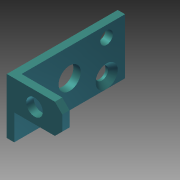
# Autodesk Inventor part: 13_0204_051
Saved by Autodesk Inventor 2012 SP1 (Build 160190100, 190)
## iProperties
Created: 2013-04-11
Part Number: 13_0204_051
Material: Default
Document SubType Name: Modeling
Designer: vogel
Density: 1 g/cm^3
Author: vogel
Autodesk Inventor part; units mm, degrees
ref_plane "YZ Plane" through (0, 0, 0) normal (1, 0, 0) x (0, 1, 0)
ref_plane "XZ Plane" through (0, 0, 0) normal (0, 1, 0) x (-1, 0, 0)
ref_plane "XY Plane" through (0, 0, 0) normal (0, 0, 1) x (1, 0, 0)
sketch "Skizze1" plane through (0, 0, 0) normal (0, 0, 1) x (1, 0, 0)
  line L0 (0, 0) -> (1.7032, 0)
  line L1 (2, 2) -> (2, 30)
  line L2 (2, 30) -> (0, 30)
  line L3 (0, 30) -> (0, 0)
  line L4 (0, 0) -> (15, 0)
  line L5 (15, 0) -> (15, 2)
  line L6 (15, 2) -> (2, 2)
  line L7 (0, 2.129) -> (0, 0)
  dimension "d0" = 30
  dimension "d1" = 15
  dimension "d2" = 2
  constraints: 16 end point, 4 parallel, 3 perpendicular, 2 horizontal
  measures "d0" distance of L2.end L0.start
  measures "d1" distance of L0.start L4.end
  measures "d2" distance of L4.end L5.end
extrude "Extrusion1" add sketch "Skizze1" along normal blind 15
sketch "Skizze2" plane through (0, 0, 0) normal (-1, 0, 0) x (0, 0, 1)
  line L0 (0, 30) -> (15, 30) projected
  line L1 (0, 0) -> (0, 30) projected
  line L2 (0, 0) -> (15, 0) projected
  line L3 (0, -6) -> (0, 36) projected
  line L4 (-3, 0) -> (18, 0) projected
  line L5 (7.5, 30) -> (7.5, 0)
  point P0 (7.5, 15)
  dimension "d5" = 30
  dimension "d6" = 7.5
  dimension "d7" = 15
  constraints: 3 midpoint, 2 end point, 1 perpendicular
  measures "d5" distance of L5.start L5.end
  measures "d6" distance between parallel lines of L5 L1
  measures "d7" distance from line of L2 point (7.5, 15)
hole "Bohrung1" at (0, 15, 7.5) direction (1, 0, 0) diameter 6 end through all
sketch "Skizze3" plane through (2, 2, 0) normal (0, 1, 0) x (1, 0, 0)
  line L0 (0, -15) -> (13, -15) projected
  line L1 (0, 0) -> (0, -15) projected
  line L2 (13, 0) -> (0, 0)
  line L3 (0, 0) -> (0, -7)
  line L4 (0, -7) -> (13, -7)
  line L5 (13, -7) -> (13, 0)
  point P0 (-2, 0)
  dimension "d15" = 8
  constraints: 8 end point, 2 parallel, 1 horizontal, 1 perpendicular, 1 point on line
  measures "d15" distance between parallel lines of L4 L0
extrude "Extrusion2" cut sketch "Skizze3" against normal through all
sketch "Skizze4" plane through (2, 0, 0) normal (1, 0, 0) x (0, 0, -1)
  line L0 (-15, 30) -> (-15, 2) projected
  line L1 (0, 30) -> (0, 0) projected
  line L2 (0, 30) -> (-15, 30) projected
  line L3 (-15, 27.5) -> (0, 27.5)
  line L4 (-15, 22) -> (0, 22)
  point P0 (-11, 25)
  point P1 (-4, 25)
  dimension "d18" = 2.5
  dimension "d19" = 8
  dimension "d20" = 5
  dimension "d21" = 5
  dimension "d22" = 4
  dimension "d23" = 4
  constraints: 4 end point, 4 point on line, 2 perpendicular
  measures "d18" distance between parallel lines of L2 L3
  measures "d19" distance between parallel lines of L2 L4
  measures "d20" distance from line of L2 point (-11, 25)
  measures "d21" distance from line of point (-4, 25) L2
  measures "d22" distance from line of point (-4, 25) L1
  measures "d23" distance from line of L0 point (-11, 25)
hole "Bohrung2" at (2, 25, 11) at (2, 25, 4) direction (-1, 0, 0) diameter 3.4 end through all
sketch "Skizze5" plane through (2, 2, 15) normal (0, 1, 0) x (1, 0, 0)
  line L0 (13, 8) -> (0, 8) projected
  line L1 (13, 8) -> (13, 0) projected
  point P0 (-2, 15)
  point P1 (5.5, 4)
  dimension "d31" = 7.5
  dimension "d32" = 4
  measures "d31" distance from line of L1 point (5.5, 4)
  measures "d32" distance from line of L0 point (5.5, 4)
hole "Bohrung3" at (7.5, 2, 11) direction (0, -1, 0) diameter 4.5 end through all
hole "Bohrung4" at (2, 25, 4) direction (-1, 0, 0) diameter 3.4 end through all countersink diameter 6 countersink angle 90
chamfer "Fase1" distance 2 angle 45 2 edges at (15, 1, 15) (15, 1, 7)
